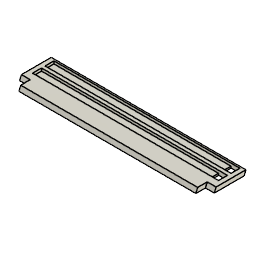
name_sign_LED_holder_top_front (Autodesk Fusion 360 design; units mm, degrees)
Autodesk Fusion 360 part; units mm, degrees
sketch "Name Sign LED Holder Top" plane through (0, 0, 0) normal (0, 1, 0) x (1, 0, 0)
  line L0 (0.5771, -64.3591) -> (5.5771, -64.3591)
  line L1 (5.5771, -64.3591) -> (5.5771, -28.5209)
  line L2 (5.5771, -28.5209) -> (36.754, -15.7343)
  line L3 (36.754, -15.7343) -> (32.9594, -6.4822)
  line L4 (32.9594, -6.4822) -> (0.5771, -19.7631)
  line L5 (0.5771, -19.7631) -> (0.5771, -64.3591)
  line L6 (0.5771, -64.3591) -> (5.5771, -62.3085)
  line L7 (32.9594, -6.4822) -> (32.9594, -17.2905)
  dimension "d1" = 5
  dimension "d2" = 10
  dimension "d3" = 112.3
  dimension "d16" = 44.596
  dimension "d18" = 22.3
  dimension "d20" = 35
  constraint horizontal L0
  constraint perpendicular L0 L1
  constraint perpendicular L2 L3
  constraint perpendicular L0 L5
  constraint parallel L2 L4
  constraint coincident L1 L6.end
  constraint parallel L2 L6
  constraint coincident L2 L7.end
  constraint vertical L7
  measures "d1" distance of L0.start L0.end
  measures "d2" distance of L2.end L3.end
  measures "d3" angle of L1 L2
  measures "d16" distance of L0.start L4.end
  measures "d18" angle of L0 L6
  measures "d20" distance of L3.end L4.end
extrude "Extrude1" add sketch "Name Sign LED Holder Top" along normal blind 220 contours L1 L2 L4 L5 L6 L7
sketch "LED Grooves" plane through (0.5771, 0, 0) normal (-1, 0, 0) x (0, -1, 0)
  line L0 (0, 19.7631) -> (0, 64.3591)
  line L1 (-220, 64.3591) -> (-220, 19.7631)
  line L2 (-220, 19.7631) -> (0, 19.7631)
  line L3 (-215, 62.3591) -> (-5, 62.3591)
  line L4 (-5, 62.3591) -> (-5, 52.3591)
  line L5 (-5, 52.3591) -> (-215, 52.3591)
  line L6 (-215, 52.3591) -> (-215, 62.3591)
  line L7 (-215, 48.3591) -> (-5, 48.3591)
  line L8 (-5, 48.3591) -> (-5, 38.3591)
  line L9 (-5, 38.3591) -> (-215, 38.3591)
  line L10 (-215, 38.3591) -> (-215, 48.3591)
  line L11 (-5, 62.3591) -> (-15, 62.3591)
  line L12 (-15, 52.3591) -> (-5, 52.3591)
  line L13 (-5, 52.3591) -> (-5, 62.3591)
  line L14 (-5, 48.3591) -> (-15, 48.3591)
  line L15 (-15, 38.3591) -> (-5, 38.3591)
  line L16 (-5, 38.3591) -> (-5, 48.3591)
  line L17 (0, 64.3591) -> (-220, 64.3591)
  dimension "d6" = 210
  dimension "d7" = 210
  dimension "d8" = 5
  dimension "d9" = 5
  dimension "d12" = 10
  dimension "d13" = 10
  dimension "d22" = 4
  dimension "d30" = 2
  constraint horizontal L3
  constraint vertical L4
  constraint horizontal L5
  constraint vertical L6
  constraint horizontal L7
  constraint vertical L8
  constraint horizontal L9
  constraint vertical L10
  constraint horizontal L11
  constraint horizontal L12
  constraint vertical L13
  constraint coincident L5 L12.start
  constraint horizontal L14
  constraint horizontal L15
  constraint vertical L16
  constraint coincident L9 L15.start
  measures "d6" distance of L3.start L3.end
  measures "d7" distance of L8.end L9.end
  measures "d8" distance of L1 L6
  measures "d9" distance of L0 L8
  measures "d12" distance of L3.start L5.end
  measures "d13" distance of L7.start L9.end
  measures "d22" distance of L5 L7
  measures "d30" distance of L3 L17
extrude "Extrude2" cut sketch "LED Grooves" against normal blind 3 contours L3 L4 L5 L6 L11 L12 L13 | L7 L8 L9 L10 L14 L15 L16
sketch "Top LED Hole" plane through (3.5771, 0, 0) normal (-1, 0, 0) x (0, -1, 0)
  line L0 (-215, 52.3591) -> (-5, 52.3591)
  line L1 (-5, 52.3591) -> (-5, 62.3591)
  line L2 (-5, 62.3591) -> (-215, 62.3591)
  line L3 (-215, 62.3591) -> (-215, 52.3591)
  line L4 (-5, 62.3591) -> (-15, 62.3591)
  line L5 (-15, 62.3591) -> (-15, 52.3591)
  line L6 (-15, 52.3591) -> (-5, 52.3591)
  line L7 (-5, 52.3591) -> (-5, 62.3591)
  dimension "d33" = 10
  dimension "d34" = 10
  constraint horizontal L4
  constraint vertical L5
  constraint horizontal L6
  constraint vertical L7
  constraint coincident L0 L5.end
  constraint coincident L1.end L2.start
  measures "d33" distance of L1.end L4.end
  measures "d34" distance of L1.end L0.end
sketch "Bottom LED Hole" plane through (3.5771, 0, 0) normal (-1, 0, 0) x (0, -1, 0)
  line L0 (-215, 38.3591) -> (-5, 38.3591)
  line L1 (-5, 38.3591) -> (-5, 48.3591)
  line L2 (-215, 48.3591) -> (-215, 38.3591)
  line L3 (-5, 48.3591) -> (-15, 48.3591)
  line L4 (-15, 48.3591) -> (-15, 38.3591)
  line L5 (-15, 38.3591) -> (-5, 38.3591)
  line L6 (-5, 38.3591) -> (-5, 48.3591)
  line L7 (-5, 48.3591) -> (-215, 48.3591)
  dimension "d26" = 10
  dimension "d27" = 10
  constraint horizontal L3
  constraint vertical L4
  constraint horizontal L5
  constraint vertical L6
  constraint coincident L0 L4.end
  constraint coincident L1.end L3.start
  measures "d26" distance of L1.end L3.end
  measures "d27" distance of L1.end L0.end
extrude "Extrude3" cut sketch "Top LED Hole" sketch "Bottom LED Hole" against normal blind 2 contours L0 L1 L2 L4 L5 L6 L7 of sketch 2 contours L0 L1 L3 L4 L5 L6 L7
sketch "Magnet Holes" plane through (7.0215, 0, 17.1201) normal (-0.379456, 0, -0.92521) x (0, -1, 0)
  line L0 (0, -28.0347) -> (0, 6.9653)
  line L1 (0, 6.9653) -> (-220, 6.9653)
  line L2 (-220, 6.9653) -> (-220, -28.0347)
  line L3 (-220, -28.0347) -> (0, -28.0347)
  circle A0 centre (-210, -5.5347) radius 2.75
  dimension "d39" = 5.5
  dimension "d47" = 10
  dimension "d48" = 12.5
  measures "d39" diameter of A0
  measures "d47" distance of L2 A0.centre
  measures "d48" distance of L1 A0.centre
extrude "Extrude4" cut sketch "Magnet Holes" against normal blind 1.5 contours A0
pattern_linear "R-Pattern1" count 4 spacing 66.6667 along (0, -1, 0) count 2 spacing 15 along (0.92521, 0, -0.379456) of "Extrude4"
sketch "Sections" plane through (0, 0, 0) normal (0, -1, 0) x (1, 0, 0)
  line L0 (0.5771, 64.3591) -> (0.5771, 19.7631)
  line L1 (0.5771, 19.7631) -> (32.9594, 6.4822)
  line L2 (32.9594, 6.4822) -> (32.9594, 17.2905)
  line L3 (32.9594, 17.2905) -> (5.5771, 28.5209)
  line L4 (5.5771, 28.5209) -> (5.5771, 62.3085)
  line L5 (5.5771, 62.3085) -> (0.5771, 64.3591)
  line L6 (5.5771, 28.5209) -> (5.5771, 17.7125)
  line L7 (5.5771, 28.5209) -> (0.5771, 30.5715)
  constraint coincident L3.end L4.start
  constraint coincident L1 L6.end
  constraint parallel L4 L6
  constraint coincident L0 L7.end
  constraint parallel L3 L7
extrude "Extrude6" cut sketch "Sections" against normal blind 220 contours L1 L2 L3 L6
extrude "Extrude7" cut sketch "Sections" against normal blind 10 from surface at -210 contours L0 L1 L6 L7
extrude "Extrude8" cut sketch "Sections" against normal blind 10 contours L0 L1 L6 L7
move_body "Move4" bodies 1 to x (0, 0, -1) y (-1, 0, 0) z (0, 1, 0) at (109.5263, 60.9932, 48.533)
move_body "Move5" bodies 1 to x (1, 0, 0) y (0, 1, 0) z (0, 0, 1) at (110.4737, -78.7061, -42.956)
equation "d4 = 200 mm + 10 mm + 5 mm + 5 mm"
equation "d6 = 200 mm + 10 mm"
equation "d7 = 200 mm + 10 mm"
equation "d16 = 50 mm - 5.404 mm"
equation "magnet_hole_diameter = 5.5 mm"
equation "magnet_hole_depth = 1.5 mm"
equation "number_of_magnet_columns = 4"
equation "number_of_magnet_rows = 2"
equation "d39 = magnet_hole_diameter"
equation "d40 = -magnet_hole_depth"
equation "d42 = number_of_magnet_columns"
equation "d43 = number_of_magnet_rows"
equation "d45 = magnet_pattern_height"
equation "magnet_hole_side_offset = 10 mm"
equation "d47 = magnet_hole_side_offset"
equation "d48 = vertical_part_width + magnet_hole_top_offset"
equation "magnet_hole_top_offset = 7.5 mm"
equation "magnet_pattern_length = 220.00 mm - 2 * ( magnet_hole_side_offset )"
equation "magnet_pattern_height = 35.00 mm - vertical_part_width - 2 * ( magnet_hole_top_offset )"
equation "vertical_part_width = 5.00 mm"
equation "support_width = 10 mm"
equation "support_tolerance = 0.2 mm"
equation "d61 = -support_width"
equation "d63 = -( 220.00 mm - support_width )"
equation "d64 = -support_width"
named bodies: "Name Sign LED Holder Top"
